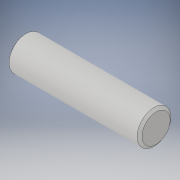
# Autodesk Inventor part: shaft 6x24-1
Saved by Autodesk Inventor 2017.1 (Build 211199000, 199)
## iProperties
Created: 2017-05-25
Part Number: shaft 6x24-1
Material: Generic
Document SubType Name: Modeling
Designer: 196918
Density: 1 g/cm^3
Appearance: Default
Author: 196918
Autodesk Inventor part; units mm, degrees
ref_plane "YZ Plane" through (0, 0, 0) normal (1, 0, 0) x (0, 1, 0)
sketch "Sketch1" plane through (0, 0, 0) normal (1, 0, 0) x (0, 1, 0)
  circle A0 centre (0, 0) radius 3.048
  dimension "d0" = 6.096
  constraints: 1 centre point, 1 coincident
  measures "d0" diameter of A0
extrude "Extrusion1" add sketch "Sketch1" along normal blind 23.114
ref_plane "Work Plane1" through (23.495, 0, 0) normal (1, 0, 0) x (0, 0, -1)
sketch "Sketch2" plane through (23.495, 0, 0) normal (1, 0, 0) x (0, 0, -1)
  circle A0 centre (0, 0) radius 2.54
  dimension "d4" = 5.08
  constraints: 1 centre point, 1 coincident
  measures "d4" diameter of A0
loft "Loft1" add profiles "Sketch2" section 2 edges at (23.114, -3.048, 0)
ref_plane "Work Plane2" through (-0.381, 0, 0) normal (-1, 0, 0) x (0, 0, 1)
sketch "Sketch3" plane through (-0.381, 0, 0) normal (-1, 0, 0) x (0, 0, 1)
  circle A0 centre (0, 0) radius 2.54
  dimension "d10" = 5.08
  constraints: 1 centre point, 1 coincident
  measures "d10" diameter of A0
loft "Loft2" add profiles "Sketch3" section 2 edges at (0, -3.048, 0)
body "Solid1"
